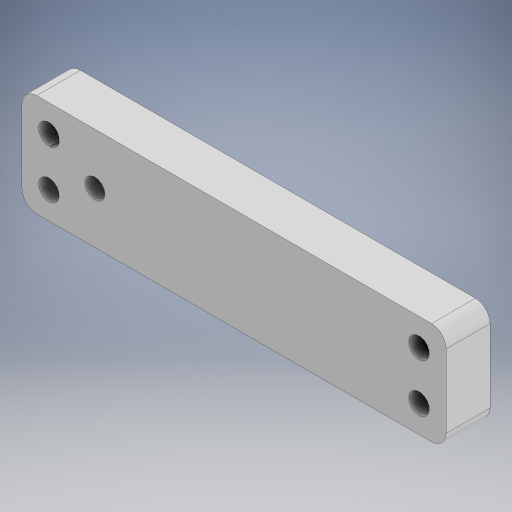
# Autodesk Inventor part: side of head_zig4
Saved by Autodesk Inventor 2024 (Build 280153000, 153)
## iProperties
Created: 2024-09-11
Part Number: side of head_zig4
Material: 일반
Document SubType Name: Modeling
Designer: ASUS
Density: 1 g/cm^3
Appearance: 기본값
Author: ASUS
Autodesk Inventor part; units mm, degrees
ref_plane "YZ Plane" through (0, 0, 0) normal (1, 0, 0) x (0, 1, 0)
ref_plane "XZ Plane" through (0, 0, 0) normal (0, 1, 0) x (-1, 0, 0)
ref_plane "XY Plane" through (0, 0, 0) normal (0, 0, 1) x (1, 0, 0)
ref_plane "작업 평면1" through (0, 0, 0) normal (0, 0, 1) x (1, 0, 0)
sketch "스케치1" plane through (0, 0, 0) normal (0, 0, 1) x (1, 0, 0)
  circle A0 centre (-44, 3) radius 1.35 projected
  line L0 (0, 0) -> (0, 6) projected
  line L1 (0, 6) -> (-50, 6) projected
  line L2 (-50, 0) -> (-50, 6) projected
  line L3 (0, 0) -> (-50, 0) projected
  line L4 (-50.3, 6.3) -> (0.3, 6.3)
  line L5 (0.3, 6.3) -> (0.3, -0.3)
  line L6 (0.3, -0.3) -> (-50.3, -0.3)
  line L7 (-50.3, -0.3) -> (-50.3, 6.3)
  line L8 (-54, 10) -> (4, 10)
  line L9 (4, 10) -> (4, -4)
  line L10 (4, -4) -> (-54, -4)
  line L11 (-54, -4) -> (-54, 10)
  dimension "d0" = 0.3
  dimension "d1" = 4
  constraints: 16 end point, 6 other
  measures "d0" distance between parallel lines of L1 L4
  measures "d1" distance between parallel lines of L1 L8
extrude "돌출1" add sketch "스케치1" along normal blind 3 contours L3 L2 L1 L0 | L4 L5 L6 L7 | L8 L9 L10 L11
sketch "스케치2" plane through (0, 0, 0) normal (0, 0, -1) x (-1, 0, 0)
  line L0 (54, -4) -> (-4, -4) projected
  line L1 (54, 10) -> (54, -4) projected
  line L2 (-4, 10) -> (54, 10) projected
  line L3 (-4, -4) -> (-4, 10) projected
  circle A0 centre (44, 3) radius 1.35 projected
  line L4 (0, 0) -> (0, 6) projected
  line L5 (50, 0) -> (50, 6) projected
  line L6 (0, 6) -> (50, 6) projected
  line L7 (0, 0) -> (50, 0) projected
  line L8 (50.3, 6.3) -> (50.3, -0.3)
  line L9 (50.3, -0.3) -> (-0.3, -0.3)
  line L10 (-0.3, -0.3) -> (-0.3, 6.3)
  line L11 (-0.3, 6.3) -> (50.3, 6.3)
  dimension "d4" = 0.3
  constraints: 8 end point, 3 other
  measures "d4" distance between parallel lines of L5 L8
extrude "돌출2" add sketch "스케치2" along normal blind 3 contours L0 L3 L2 L1
sketch "스케치3" plane through (0, 0, -3) normal (0, 0, -1) x (-1, 0, 0)
  line L0 (54, 10) -> (-4, 10) projected
  line L1 (-4, 10) -> (-4, -4) projected
  line L2 (-4, -4) -> (54, -4) projected
  line L3 (54, -4) -> (54, 10) projected
  line L4 (50.3, 6.3) -> (50.3, -0.3) projected
  line L5 (50.3, -0.3) -> (-0.3, -0.3) projected
  line L6 (-0.3, -0.3) -> (-0.3, 6.3) projected
  line L7 (-0.3, 6.3) -> (50.3, 6.3) projected
  point P0 (0, 0)
hole "구멍1" at (-50.3, -0.3, -3) at (-50.3, 6.3, -3) at (0.3, -0.3, -3) at (0.3, 6.3, -3) direction (0, 0, 1) diameter 3.2 end through all
fillet "모깎기1" radius 2 4 edges at (-54, 10, 0) (-54, -4, 0) (4, -4, 0) (4, 10, 0)
sketch "스케치4" plane through (0, 0, -3) normal (0, 0, -1) x (-1, 0, 0)
  arc A0 (1.3, 6.3) -> (-0.3, 4.7) centre (-0.3, 6.3) ccw projected
  line L0 (1.3, 6.3) -> (48.7, 6.3) projected
  arc A1 (50.3, 4.7) -> (48.7, 6.3) centre (50.3, 6.3) ccw projected
  line L1 (50.3, 4.7) -> (50.3, 1.3) projected
  arc A2 (48.7, -0.3) -> (50.3, 1.3) centre (50.3, -0.3) ccw projected
  line L2 (48.7, -0.3) -> (1.3, -0.3) projected
  arc A3 (-0.3, 1.3) -> (1.3, -0.3) centre (-0.3, -0.3) ccw projected
  line L3 (-0.3, 1.3) -> (-0.3, 4.7) projected
  arc A4 (-2, 10) -> (-4, 8) centre (-2, 8) ccw projected
  line L4 (-4, 8) -> (-4, -2) projected
  arc A5 (-4, -2) -> (-2, -4) centre (-2, -2) ccw projected
  line L5 (-2, -4) -> (52, -4) projected
  arc A6 (52, -4) -> (54, -2) centre (52, -2) ccw projected
  line L6 (54, -2) -> (54, 8) projected
  arc A7 (54, 8) -> (52, 10) centre (52, 8) ccw projected
  line L7 (52, 10) -> (-2, 10) projected
  line L8 (1.0856, -0.1) -> (48.9144, -0.1)
  arc A8 (48.9144, -0.1) -> (50.1, 1.0856) centre (50.3, -0.3) ccw
  line L9 (50.1, 1.0856) -> (50.1, 4.9144)
  arc A9 (50.1, 4.9144) -> (48.9144, 6.1) centre (50.3, 6.3) ccw
  line L10 (48.9144, 6.1) -> (1.0856, 6.1)
  arc A10 (1.0856, 6.1) -> (-0.1, 4.9144) centre (-0.3, 6.3) ccw
  line L11 (-0.1, 4.9144) -> (-0.1, 1.0856)
  arc A11 (-0.1, 1.0856) -> (1.0856, -0.1) centre (-0.3, -0.3) ccw
  point P0 (0, 0)
  dimension "d15" = 0.2
  constraints: 8 end point, 8 point on circle, 4 centre point, 7 other
  measures "d15" distance between parallel lines of L2 L8
extrude "돌출3" add sketch "스케치4" against normal up to surface (6 mm away) contours L0 A1 L1 A2 L2 A3 L3 A0
sketch "스케치5" plane through (0, 0, 0) normal (0, 0, -1) x (-1, 0, 0)
  arc A0 (-0.1, 1.0856) -> (1.0856, -0.1) centre (-0.3, -0.3) ccw projected
  line L0 (-0.1, 1.0856) -> (-0.1, 4.9144) projected
  arc A1 (1.0856, 6.1) -> (-0.1, 4.9144) centre (-0.3, 6.3) ccw projected
  line L1 (1.0856, 6.1) -> (48.9144, 6.1) projected
  arc A2 (50.1, 4.9144) -> (48.9144, 6.1) centre (50.3, 6.3) ccw projected
  line L2 (50.1, 4.9144) -> (50.1, 1.0856) projected
  arc A3 (48.9144, -0.1) -> (50.1, 1.0856) centre (50.3, -0.3) ccw projected
  line L3 (48.9144, -0.1) -> (1.0856, -0.1) projected
  arc A4 (-2, 10) -> (-4, 8) centre (-2, 8) ccw projected
  line L4 (-4, 8) -> (-4, -2) projected
  arc A5 (-4, -2) -> (-2, -4) centre (-2, -2) ccw projected
  line L5 (-2, -4) -> (52, -4) projected
  arc A6 (52, -4) -> (54, -2) centre (52, -2) ccw projected
  line L6 (54, -2) -> (54, 8) projected
  arc A7 (54, 8) -> (52, 10) centre (52, 8) ccw projected
  line L7 (52, 10) -> (-2, 10) projected
  arc A8 (50.1, 1.2875) -> (48.7125, -0.1) centre (50.3, -0.3) ccw projected
  circle A9 centre (50.3, -0.3) radius 1.4
  circle A10 centre (50.3, 6.3) radius 1.45
  circle A11 centre (-0.3, 6.3) radius 1.4
  arc A12 (1.2875, -0.1) -> (-0.1, 1.2875) centre (-0.3, -0.3) ccw projected
  circle A13 centre (-0.3, -0.3) radius 1.4
  line L8 (50.1, 1.2875) -> (50.1, 4.7125) projected
  arc A14 (48.7125, 6.1) -> (50.1, 4.7125) centre (50.3, 6.3) ccw projected
  line L9 (48.7125, 6.1) -> (1.2875, 6.1) projected
  arc A15 (-0.1, 4.7125) -> (1.2875, 6.1) centre (-0.3, 6.3) ccw projected
  line L10 (-0.1, 4.7125) -> (-0.1, 1.2875) projected
  arc A16 (1.2875, -0.1) -> (-0.1, 1.2875) centre (-0.3, -0.3) ccw projected
  line L11 (1.2875, -0.1) -> (48.7125, -0.1) projected
  arc A17 (50.1, 1.2875) -> (48.7125, -0.1) centre (50.3, -0.3) ccw projected
  circle A18 centre (44, 3) radius 1.35 projected
  point P0 (0, 0)
  point P1 (48.7125, 6.1)
  point P2 (50.1, 4.8639)
  point P3 (48.8639, 6.1)
  point P4 (50.1, 1.0856)
  point P5 (1.0856, 6.1)
  point P6 (-0.1, 4.9144)
  constraints: 4 coincident, 2 centre point, 1 concentric, 6 other
extrude "돌출4" add sketch "스케치5" against normal up to surface (3 mm away) contours L0 A12 L3 A13 | L0 A11 L1 A15 | A8 L2 A9 L3 | L1 A10 L2 A14
